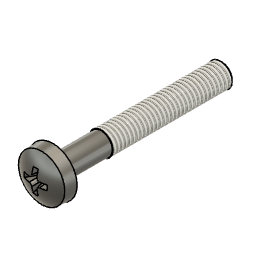
33d5ddd1-caff-4612-bc88-985aade7abc6 (Autodesk Fusion 360 design; units mm, degrees)
description: Raised Cheese Head Screw DIN 7985 - M5 x 35 - H
Autodesk Fusion 360 part; units mm, degrees
sketch "Sketch1" plane through (0, 0, 0) normal (0, 1, 0) x (1, 0, 0)
  line L0 (-2.5, 35) -> (0, 35)
  line L1 (0, 35) -> (0, -3.95)
  line L2 (-2.3, 0) -> (-5, 0)
  line L3 (-5, 0) -> (-4.794, -2.3545)
  arc A0 (-4.794, -2.3545) -> (0, -3.95) centre (0, 4.05) ccw
  line L4 (-2.3, 0) -> (-2.3, 10)
  line L5 (-2.3, 10) -> (-2.5, 10)
  line L6 (-2.5, 10) -> (-2.5, 35)
  dimension "d66" = 10
  dimension "d67" = 3.95
  dimension "d68" = 35
  dimension "d70" = 8
  dimension "d79" = 5
  dimension "d81" = 4.6
  dimension "d84" = 10
  dimension "d85" = 85
  constraint collinear origin L1.end L0.end
  constraint coincident origin L2
  constraint vertical L1
  constraint coincident L1 A0.centre
  constraint perpendicular L2 L4
  constraint perpendicular L4 L5
  constraint perpendicular L0 L6
  constraint coincident L0.start L6.end
  constraint vertical L6
  constraint vertical L4
  measures "d67" vertical distance of L1.end L2.end
  measures "d68" distance of origin L0.end
  measures "d70" radius of A0
  measures "d84" distance of L2 L5
  measures "d85" angle of L2 L3
revolve "Revolve1" add sketch "Sketch1" angle 360 about axis through (0, 0, -35) along (0, 0, 1) makes body 1
ref_plane "WorkPlane1" through (0, 0, 3.95) normal (0, 0, 1) x (1, 0, 0)
sketch "Sketch2" plane through (0, 0, 3.95) normal (0, 0, 1) x (1, 0, 0)
  line L0 (-0.53, 2.65) -> (-0.53, 0.53)
  line L1 (-0.53, 0.53) -> (-2.65, 0.53)
  line L2 (0, 0) -> (0, 2.65) construction
  line L3 (0.53, 0.53) -> (2.65, 0.53)
  line L4 (0.53, 2.65) -> (0.53, 0.53)
  line L5 (0.53, -0.53) -> (2.65, -0.53)
  line L6 (0.53, -2.65) -> (0.53, -0.53)
  line L7 (-0.53, -2.65) -> (-0.53, -0.53)
  line L8 (-0.53, -0.53) -> (-2.65, -0.53)
  line L9 (-0.53, 2.65) -> (0.53, 2.65)
  line L10 (-2.65, 0.53) -> (-2.65, -0.53)
  line L11 (-0.53, -2.65) -> (0.53, -2.65)
  line L12 (2.65, -0.53) -> (2.65, 0.53)
  line L13 (-2.65, 0) -> (2.65, 0) construction
  dimension "d22" = 1.06
  dimension "d57" = 5.3
  dimension "d99" = 5.3
  constraint perpendicular L0 L1
  constraint symmetric L0.start L2 L4.start
  constraint symmetric L0.end L2 L3.start
  constraint symmetric L1.end L2 L3.end
  constraint perpendicular L4 L9
  constraint perpendicular L8 L10
  constraint equal L9 L10
  constraint equal L0 L1
  constraint horizontal L0.start L2.end
  constraint vertical L2
  constraint collinear L4 L6
  constraint midpoint L10 L13.start
  constraint midpoint L12 L13.end
  constraint perpendicular L12 L13
  constraint coincident L2.start L13
  constraint horizontal L8
  constraint horizontal L5
  constraint horizontal L11
  constraint coincident origin L2
  measures "d22" horizontal distance of L0.start L4.start
  measures "d57" distance of L10 L12
  measures "d99" distance of L9 L11
extrude "Extrude1" add sketch "Sketch2" against normal blind 2 draft -4 separate body makes body 2
draft "Draft1" angle -30 neutral plane through (0, 0, 3.95) pull (0, 0, 1) 4 faces at (2.6034, 0.13, 3.2833) (0.13, 2.6034, 3.2833) (-2.6034, 0.13, 3.2833) (0.13, -2.6034, 3.2833) on bodies 2
fillet "Fillet3" radius 0.53 4 edges at (-0.4601, 0.4601, 2.95) (0.4601, 0.4601, 2.95) (0.4601, -0.4601, 2.95) (-0.4601, -0.4601, 2.95) on bodies 2
combine "Combine1" operation cut target body 1 tool bodies 2
thread "Thread2" "ISO Metric profile 5.0 M5x0.8 6g" major diameter 4.901 minor diameter 3.9895 pitch 0.8 angle 60 resizes the face on face at (-2.4969, 0.1246, -18.3333) on bodies 1
sketch "Sketch5" plane through (0, 0, 0) normal (0, 1, 0) x (1, 0, 0)
  line L0 (0, 35) -> (0, -3.95)
  line L1 (0, 35) -> (-2.55, 35)
  line L2 (-2.55, 35) -> (-2.55, 34.6)
  line L3 (-2.55, 34.6) -> (-2.15, 35)
  dimension "d93" = 45
  dimension "d94" = 2.15
  dimension "d95" = 2.55
  constraint coincident L0.start L1.start
  constraint perpendicular L0 L1
  constraint perpendicular L1 L2
  constraint coincident L1 L3.end
  measures "d93" angle of L2 L3
  measures "d94" horizontal distance of origin L3.end
  measures "d95" horizontal distance of origin L1.end
revolve "Revolve2" cut sketch "Sketch5" angle 360 about axis through (0, 0, 1.75) along (0, 0, 1) bodies 1
equation "adsk_nomlen = 35.00 mm"
equation "adsk_headh = 3.95 mm"
equation "adsk_headdia = 10.00 mm"
equation "adsk_nomdia = 5.00 mm"
equation "d22 = adsk_philwidth"
equation "adsk_phildia = 5.30 mm"
equation "d31 = -adsk_phildepth"
equation "adsk_phildepth = 2.00 mm"
equation "d57 = adsk_phildia"
equation "d59 = adsk_phildia * 0.1"
equation "d66 = adsk_headdia"
equation "d67 = adsk_headh"
equation "d68 = adsk_nomlen"
equation "d70 = adsk_headdia * 0.8"
equation "d71 = adsk_headh"
equation "adsk_thrlen = 25.00 mm"
equation "d79 = adsk_nomdia"
equation "d81 = adsk_nomdia - ( adsk_pitch1 / 2 )"
equation "adsk_pitch1 = 0.80 mm"
equation "d84 = adsk_nomlen - adsk_thrlen"
equation "d94 = d95 - ( adsk_pitch1 / 2 )"
equation "d95 = adsk_nomdia * 0.51"
equation "adsk_philwidth = adsk_phildia / 5"
equation "d99 = adsk_phildia"
